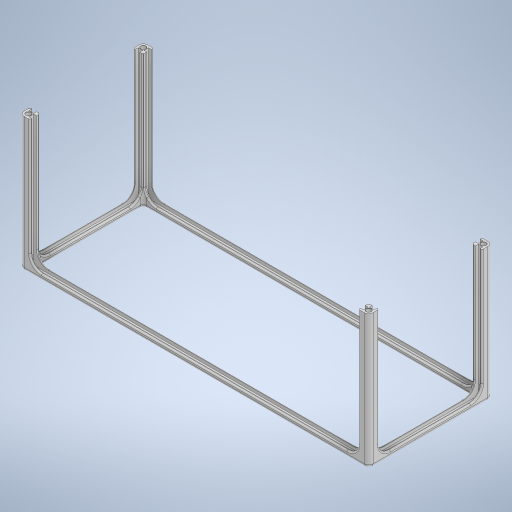
# Autodesk Inventor part: ChamberFrameBottom
Saved by Autodesk Inventor 2023 (Build 270158000, 158)
## iProperties
Created: 2025-11-21
Part Number: ChamberFrameBottom
Material: Generic
Document SubType Name: Modeling
Designer: DanAr
Density: 1 g/cm^3
Appearance: Default
Author: DanAr
Autodesk Inventor part; units mm, degrees
ref_plane "YZ Plane" through (0, 0, 0) normal (1, 0, 0) x (0, 1, 0)
ref_plane "XZ Plane" through (0, 0, 0) normal (0, 1, 0) x (-1, 0, 0)
ref_plane "XY Plane" through (0, 0, 0) normal (0, 0, 1) x (1, 0, 0)
sketch "Sketch1" plane through (0, 0, 0) normal (0, 1, 0) x (-1, 0, 0)
  line L0 (0, 0) -> (234, 0)
  line L1 (234, 0) -> (234, -79)
  line L2 (234, -79) -> (0, -79)
  line L3 (0, -79) -> (0, 0)
  line L4 (2, -77.5) -> (232, -77.5)
  line L5 (232, -77.5) -> (232, -80.5)
  line L6 (232, -80.5) -> (2, -80.5)
  line L7 (2, -80.5) -> (2, -77.5)
  line L8 (2, -77.5) -> (232, -80.5) construction
  line L9 (232, -77.5) -> (2, -80.5) construction
  line L10 (235.5, -2) -> (232.5, -2)
  line L11 (232.5, -2) -> (232.5, -77)
  line L12 (232.5, -77) -> (235.5, -77)
  line L13 (235.5, -77) -> (235.5, -2)
  line L14 (235.5, -2) -> (232.5, -77) construction
  line L15 (232.5, -2) -> (235.5, -77) construction
  line L16 (1.5, -2) -> (-1.5, -2)
  line L17 (-1.5, -2) -> (-1.5, -77)
  line L18 (-1.5, -77) -> (1.5, -77)
  line L19 (1.5, -77) -> (1.5, -2)
  line L20 (1.5, -2) -> (-1.5, -77) construction
  line L21 (-1.5, -2) -> (1.5, -77) construction
  line L22 (2, 1.5) -> (232, 1.5)
  line L23 (232, 1.5) -> (232, -1.5)
  line L24 (232, -1.5) -> (2, -1.5)
  line L25 (2, -1.5) -> (2, 1.5)
  line L26 (2, 1.5) -> (232, -1.5) construction
  line L27 (232, 1.5) -> (2, -1.5) construction
  line L28 (117, 0) -> (117, -79)
  line L29 (231, -3) -> (3, -3)
  line L30 (3, -3) -> (3, -76)
  line L31 (3, -76) -> (231, -76)
  line L32 (231, -76) -> (231, -3)
  line L33 (231, -3) -> (3, -76) construction
  line L34 (3, -3) -> (231, -76) construction
  line L35 (-3, 3) -> (237, 3)
  line L36 (237, 3) -> (237, -82)
  line L37 (237, -82) -> (-3, -82)
  line L38 (-3, -82) -> (-3, 3)
  line L39 (-3, 3) -> (237, -82) construction
  line L40 (237, 3) -> (-3, -82) construction
  point P0 (234, -39.5)
  point P1 (0, -39.5)
  point P2 (117, -39.5)
  dimension "d0" = 79
  dimension "d1" = 234
  dimension "d2" = 230
  dimension "d3" = 3
  dimension "d4" = 75
  dimension "d5" = 3
  dimension "d6" = 75
  dimension "d7" = 3
  dimension "d8" = 230
  dimension "d9" = 3
  dimension "d10" = 73
  dimension "d11" = 228
  dimension "d12" = 240
  dimension "d13" = 85
  constraints: 82 end point, 17 midpoint, 14 parallel, 8 perpendicular, 7 horizontal
  measures "d0" distance of L0.end L1.end
  measures "d1" distance of L1.end L2.end
  measures "d2" distance of L5.end L6.end
  measures "d3" distance of L4.end L5.end
  measures "d4" distance of L12.end L10.start
  measures "d5" distance of L11.end L12.end
  measures "d6" distance of L18.end L16.start
  measures "d7" distance of L17.end L18.end
  measures "d8" horizontal distance of L22.end L24.end
  measures "d9" distance of L22.end L23.end
  measures "d10" distance of L29.end L30.end
  measures "d11" distance of L30.end L31.end
  measures "d12" distance of L36.end L37.end
  measures "d13" distance of L37.end L35.start
extrude "Extrusion1" add sketch "Sketch1" along normal blind 4 contours L0 L25 L24 L28 L29 L30 L31 L4 L7 L2 L3 L18 L19 L16 | L0 L1 L10 L11 L12 L2 L5 L4 L28 L31 L32 L29 L24 L23 | L35 L36 L37 L38
sketch "Sketch2" plane through (0, 0, 0) normal (0, -1, 0) x (1, 0, 0)
  line L0 (3, 3) -> (3, -82) projected
  line L1 (3, -82) -> (-237, -82) projected
  line L2 (3, 3) -> (-237, 3)
  line L3 (-237, 3) -> (-237, -82)
  line L4 (-237, -82) -> (3, -82)
  line L5 (3, -82) -> (3, 3)
  line L6 (-3, -76) -> (-3, -3) projected
  line L7 (-231, -3) -> (-231, -76) projected
  line L8 (-3, -3) -> (-231, -3)
  line L9 (-231, -3) -> (-231, -76)
  line L10 (-231, -76) -> (-3, -76)
  line L11 (-3, -76) -> (-3, -3)
  point P0 (0, 0)
  point P1 (-231, -3)
  point P2 (-3, -76)
  constraints: 16 end point, 4 parallel, 2 horizontal, 2 perpendicular
extrude "Extrusion2" add sketch "Sketch2" against normal blind 2
sketch "Sketch3" plane through (0, 4, 0) normal (0, 1, 0) x (1, 0, 0)
  line L0 (-1.5, 2) -> (-1.5, 77) projected
  line L1 (1.5, 77) -> (1.5, 2) projected
  line L2 (-1.5, 2) -> (1.5, 2)
  line L3 (1.5, 2) -> (1.5, 4)
  line L4 (1.5, 4) -> (-1.5, 4)
  line L5 (-1.5, 4) -> (-1.5, 2)
  line L6 (-232, 1.5) -> (-2, 1.5) projected
  line L7 (-2, -1.5) -> (-232, -1.5) projected
  line L8 (-2, 1.5) -> (-4, 1.5)
  line L9 (-4, 1.5) -> (-4, -1.5)
  line L10 (-4, -1.5) -> (-2, -1.5)
  line L11 (-2, -1.5) -> (-2, 1.5)
  line L12 (-3, 76) -> (-3, 3) projected
  line L13 (-4, 1.5) -> (-3, 1.5)
  line L14 (-3, 3) -> (-4, 3)
  line L15 (-4, 3) -> (-4, 1.5)
  line L16 (-3, 3) -> (-231, 3) projected
  line L17 (-1.5, 3) -> (-1.5, 4)
  line L18 (-1.5, 4) -> (-3, 4)
  line L19 (-3, 4) -> (-3, 3)
  line L20 (-237, -3) -> (3, -3) projected
  line L21 (3, -1.5) -> (3, -3)
  line L22 (3, -3) -> (-4, -3)
  line L23 (-4, -3) -> (-4, -1.5)
  line L24 (1.5, 4) -> (3, 4)
  line L25 (3, 4) -> (3, -1.5)
  line L26 (-1.5, 77) -> (1.5, 77) projected
  line L27 (-1.5, 77) -> (1.5, 77)
  line L28 (1.5, 77) -> (1.5, 75)
  line L29 (1.5, 75) -> (-1.5, 75)
  line L30 (-1.5, 75) -> (-1.5, 77)
  line L31 (-2, 77.5) -> (-232, 77.5) projected
  line L32 (-232, 80.5) -> (-2, 80.5) projected
  line L33 (-2, 77.5) -> (-4, 77.5)
  line L34 (-4, 77.5) -> (-4, 80.5)
  line L35 (-4, 80.5) -> (-2, 80.5)
  line L36 (-2, 80.5) -> (-2, 77.5)
  line L37 (-231, 76) -> (-3, 76) projected
  line L38 (-4, 77.5) -> (-3, 77.5)
  line L39 (-3, 76) -> (-4, 76)
  line L40 (-4, 76) -> (-4, 77.5)
  line L41 (-1.5, 75) -> (-3, 75)
  line L42 (-3, 75) -> (-3, 76)
  line L43 (-1.5, 76) -> (-1.5, 75)
  line L44 (3, 82) -> (-237, 82) projected
  line L45 (1.5, 75) -> (3, 75)
  line L46 (3, 75) -> (3, 82)
  line L47 (3, 82) -> (1.5, 82)
  line L48 (1.5, 82) -> (-4, 82)
  line L49 (-4, 82) -> (-4, 80.5)
  line L50 (-232, 77.5) -> (-230, 77.5)
  line L51 (-230, 77.5) -> (-230, 80.5)
  line L52 (-230, 80.5) -> (-232, 80.5)
  line L53 (-232, 80.5) -> (-232, 77.5)
  line L54 (-235.5, 2) -> (-235.5, 77) projected
  line L55 (-232.5, 77) -> (-232.5, 2) projected
  line L56 (-235.5, 77) -> (-232.5, 77)
  line L57 (-232.5, 77) -> (-232.5, 75)
  line L58 (-232.5, 75) -> (-235.5, 75)
  line L59 (-235.5, 75) -> (-235.5, 77)
  line L60 (-232.5, 75) -> (-231, 75)
  line L61 (-231, 75) -> (-231, 76)
  line L62 (-232.5, 39) -> (-232.5, 75)
  line L63 (-230, 77.5) -> (-231, 77.5)
  line L64 (-231, 76) -> (-230, 76)
  line L65 (-230, 76) -> (-230, 77.5)
  line L66 (-237, 82) -> (-237, -3) projected
  line L67 (-237, 80.5) -> (-237, 82)
  line L68 (-237, 82) -> (-230, 82)
  line L69 (-230, 82) -> (-230, 80.5)
  line L70 (-235.5, 75) -> (-237, 75)
  line L71 (-237, 75) -> (-237, 80.5)
  line L72 (-232.5, 2) -> (-235.5, 2) projected
  line L73 (-232.5, 2) -> (-235.5, 2)
  line L74 (-235.5, 2) -> (-235.5, 4)
  line L75 (-235.5, 4) -> (-232.5, 4)
  line L76 (-232.5, 4) -> (-232.5, 2)
  line L77 (-232, -1.5) -> (-232, 1.5) projected
  line L78 (-232, 1.5) -> (-230, 1.5)
  line L79 (-230, 1.5) -> (-230, -1.5)
  line L80 (-230, -1.5) -> (-232, -1.5)
  line L81 (-232, -1.5) -> (-232, 1.5)
  line L82 (-232.5, 4) -> (-231, 4)
  line L83 (-231, 4) -> (-231, 3)
  line L84 (-232.5, 3) -> (-232.5, 4)
  line L85 (-231, 3) -> (-230, 3)
  line L86 (-230, 3) -> (-230, 1.5)
  line L87 (-230, 1.5) -> (-231, 1.5)
  line L88 (-237, -1.5) -> (-237, -3)
  line L89 (-237, -3) -> (-230, -3)
  line L90 (-230, -3) -> (-230, -1.5)
  line L91 (-235.5, 4) -> (-237, 4)
  line L92 (-237, 4) -> (-237, -1.5)
  point P0 (0, 0)
  point P1 (-2, 80.5)
  point P2 (-1.5, 75)
  point P3 (1.5, 2)
  point P4 (-2, -1.5)
  dimension "d18" = 2
  dimension "d19" = 2
  dimension "d20" = 2
  dimension "d21" = 2
  dimension "d22" = 2
  dimension "d23" = 2
  dimension "d24" = 2
  dimension "d25" = 2
  constraints: 152 end point, 28 parallel, 17 horizontal, 14 perpendicular, 8 point on line
  measures "d18" distance between parallel lines of L2 L4
  measures "d19" distance between parallel lines of L11 L9
  measures "d20" distance between parallel lines of L27 L29
  measures "d21" distance between parallel lines of L36 L34
  measures "d22" distance between parallel lines of L53 L51
  measures "d23" distance between parallel lines of L56 L58
  measures "d24" distance between parallel lines of L72 L75
  measures "d25" distance between parallel lines of L77 L79
extrude "Extrusion3" add sketch "Sketch3" along normal blind 178 contours L2 L1 L24 L25 L21 L20 L23 L7 L11 L6 L15 L14 L12 L18 L0 | L41 L12 L37 L40 L31 L36 L32 L49 L44 L46 L45 L1 L26 L0 | L86 L6 L77 L7 L90 L20 L66 L91 L54 L72 L55 L82 L83 L16 | L37 L61 L60 L55 L56 L54 L70 L66 L44 L69 L32 L53 L31 L65
sketch "Sketch4" plane through (0, 182, 0) normal (0, 1, 0) x (1, 0, 0)
  line L0 (-231, 3) -> (-231, 76) projected
  line L1 (-3, 76) -> (-3, 3) projected
  line L2 (-231, 76) -> (-3, 76)
  line L3 (-3, 76) -> (-3, 3)
  line L4 (-3, 3) -> (-231, 3)
  line L5 (-231, 3) -> (-231, 76)
  line L6 (3, -3) -> (3, 82) projected
  line L7 (-237, 82) -> (-237, -3) projected
  line L8 (3, -3) -> (-237, -3)
  line L9 (-237, -3) -> (-237, 82)
  line L10 (-237, 82) -> (3, 82)
  line L11 (3, 82) -> (3, -3)
  line L12 (-231, 76) -> (-3, 76) projected
  line L13 (-117, 76) -> (-117, 3)
  line L14 (-4, 3) -> (-230, 3) projected
  line L15 (-2, 2) -> (-232, 2)
  line L16 (-232, 2) -> (-232, 77)
  line L17 (-232, 77) -> (-2, 77)
  line L18 (-2, 77) -> (-2, 2)
  line L19 (-2, 2) -> (-232, 77) construction
  line L20 (-232, 2) -> (-2, 77) construction
  point P0 (0, 0)
  point P1 (-117, 39.5)
  point P2 (-231, 3)
  point P3 (-3, 76)
  dimension "d28" = 75
  dimension "d29" = 230
  constraints: 30 end point, 6 parallel, 5 midpoint, 3 horizontal, 3 perpendicular
  measures "d28" distance of L15.end L16.end
  measures "d29" distance of L16.end L17.end
extrude "Extrusion4" add sketch "Sketch4" along normal blind 0.5 contours L15 L16 L17 L18
sketch "Sketch5" plane through (0, 182, 0) normal (0, 1, 0) x (1, 0, 0)
  line L0 (-1.5, 2) -> (-1.5, 4) projected
  line L1 (-1.5, 77) -> (1.5, 77) projected
  line L2 (-1.5, 2) -> (1.5, 2)
  line L3 (1.5, 2) -> (1.5, 77)
  line L4 (1.5, 77) -> (-1.5, 77)
  line L5 (-1.5, 77) -> (-1.5, 2)
  line L6 (-2, 77.5) -> (-232, 77.5) projected
  line L7 (-232, 80.5) -> (-230, 80.5) projected
  line L8 (-2, 77.5) -> (-232, 77.5)
  line L9 (-232, 77.5) -> (-232, 80.5)
  line L10 (-232, 80.5) -> (-2, 80.5)
  line L11 (-2, 80.5) -> (-2, 77.5)
  line L12 (-235.5, 75) -> (-235.5, 77) projected
  line L13 (-232.5, 2) -> (-235.5, 2) projected
  line L14 (-235.5, 77) -> (-232.5, 77)
  line L15 (-232.5, 77) -> (-232.5, 2)
  line L16 (-232.5, 2) -> (-235.5, 2)
  line L17 (-235.5, 2) -> (-235.5, 77)
  line L18 (-232, 1.5) -> (-230, 1.5) projected
  line L19 (-2, 1.5) -> (-2, -1.5) projected
  line L20 (-232, 1.5) -> (-2, 1.5)
  line L21 (-2, 1.5) -> (-2, -1.5)
  line L22 (-2, -1.5) -> (-232, -1.5)
  line L23 (-232, -1.5) -> (-232, 1.5)
  line L24 (-237, -3) -> (3, -3) projected
  line L25 (-230, 82) -> (-237, 82) projected
  line L26 (3, -3) -> (-237, -3)
  line L27 (-237, -3) -> (-237, 82)
  line L28 (-237, 82) -> (3, 82)
  line L29 (3, 82) -> (3, -3)
  line L30 (-2, 77) -> (-232, 77) projected
  line L31 (-2, 2) -> (-2, 77) projected
  line L32 (-232, 77) -> (-2, 77)
  line L33 (-2, 77) -> (-2, 2)
  line L34 (-2, 2) -> (-232, 2)
  line L35 (-232, 2) -> (-232, 77)
  point P0 (0, 0)
  point P1 (-2, 1.5)
  constraints: 48 end point, 12 parallel, 6 horizontal, 6 perpendicular
extrude "Extrusion5" add sketch "Sketch5" along normal blind 2
sketch "Sketch6" plane through (0, 184, 0) normal (0, 1, 0) x (1, 0, 0)
  line L0 (-237, -3) -> (3, -3) projected
  line L1 (-232, 2) -> (-2, 2) projected
  line L2 (3, -3) -> (-2, -3)
  line L3 (-2, -3) -> (-2, 2)
  line L4 (-2, 2) -> (3, 2)
  line L5 (3, 2) -> (3, -3)
  circle A0 centre (0, 0) radius 1.45
  circle A1 centre (0, 79) radius 1.45
  line L6 (-232.5, 2) -> (-235.5, 2) projected
  line L7 (-234, 2) -> (-234, 0)
  line L8 (-234, 0) -> (-234, 79)
  circle A2 centre (-234, 79) radius 1.45
  circle A3 centre (-234, 0) radius 1.45
  line L9 (-237, 82) -> (-237, -3) projected
  line L10 (-234, 0) -> (-237, 0)
  line L11 (-237, 0) -> (-237, -3)
  line L12 (-237, -3) -> (-234, -3)
  line L13 (-234, -3) -> (-234, 0)
  line L14 (0, 79) -> (0, 0)
  dimension "d34" = 2.9
  dimension "d57" = 3
  dimension "d58" = 79
  dimension "d59" = 3
  dimension "d60" = 79
  constraints: 22 end point, 4 centre point, 4 parallel, 3 coincident, 2 horizontal, 2 perpendicular, 2 vertical, 1 midpoint, 1 point on line
  measures "d34" diameter of A0
  measures "d57" distance of L10.end L0.start
  measures "d58" distance of L7.end L8.end
  measures "d59" distance from line of L0 point (0, 0)
  measures "d60" distance of L14.start L14.end
extrude "Extrusion6" cut sketch "Sketch6" against normal blind 20 contours L13 L7 A3 | A3 L10 L13 | A3 L7 L10 | A0 | A1 | A2
fillet "Fillet1" radius 3 4 edges at (-237, 92, 3) (-237, 92, -82) (3, 92, 3) (3, 92, -82)
chamfer "Chamfer1" distance 0.2 angle 45 4 edges at (-235.45, 184, -79) (-235.45, 184, 0) (-1.45, 184, -79) (-1.45, 184, 0)
sketch "Sketch9" plane through (0, 182, 0) normal (0, -1, 0) x (1, 0, 0)
  line L0 (-230, 3) -> (-4, 3) projected
  line L1 (-4, 1.5) -> (-230, 1.5) projected
  line L2 (-230, 3) -> (-4, 3)
  line L3 (-4, 3) -> (-4, 1.5)
  line L4 (-4, 1.5) -> (-230, 1.5)
  line L5 (-230, 1.5) -> (-230, 3)
  line L6 (-4, -1.5) -> (-4, -3) projected
  line L7 (-230, -1.5) -> (-230, -3) projected
  line L8 (-4, -1.5) -> (-230, -1.5)
  line L9 (-230, -1.5) -> (-230, -3)
  line L10 (-230, -3) -> (-4, -3)
  line L11 (-4, -3) -> (-4, -1.5)
  line L12 (-232.5, -4) -> (-231, -4) projected
  line L13 (-231, -75) -> (-232.5, -75) projected
  line L14 (-232.5, -4) -> (-231, -4)
  line L15 (-231, -4) -> (-231, -75)
  line L16 (-231, -75) -> (-232.5, -75)
  line L17 (-232.5, -75) -> (-232.5, -4)
  line L18 (-235.5, -75) -> (-237, -75) projected
  line L19 (-237, -4) -> (-235.5, -4) projected
  line L20 (-235.5, -75) -> (-237, -75)
  line L21 (-237, -75) -> (-237, -4)
  line L22 (-237, -4) -> (-235.5, -4)
  line L23 (-235.5, -4) -> (-235.5, -75)
  line L24 (-230, -77.5) -> (-230, -76) projected
  line L25 (-4, -76) -> (-4, -77.5) projected
  line L26 (-230, -76) -> (-4, -76)
  line L27 (-4, -76) -> (-4, -77.5)
  line L28 (-4, -77.5) -> (-230, -77.5)
  line L29 (-230, -77.5) -> (-230, -76)
  line L30 (-4, -80.5) -> (-4, -82) projected
  line L31 (-230, -82) -> (-230, -80.5) projected
  line L32 (-4, -80.5) -> (-230, -80.5)
  line L33 (-230, -80.5) -> (-230, -82)
  line L34 (-230, -82) -> (-4, -82)
  line L35 (-4, -82) -> (-4, -80.5)
  line L36 (-1.5, -75) -> (-3, -75) projected
  line L37 (-3, -4) -> (-1.5, -4) projected
  line L38 (-3, -75) -> (-1.5, -75)
  line L39 (-1.5, -75) -> (-1.5, -4)
  line L40 (-1.5, -4) -> (-3, -4)
  line L41 (-3, -4) -> (-3, -75)
  line L42 (3, -4) -> (1.5, -4) projected
  line L43 (1.5, -75) -> (3, -75) projected
  line L44 (1.5, -4) -> (3, -4)
  line L45 (3, -4) -> (3, -75)
  line L46 (3, -75) -> (1.5, -75)
  line L47 (1.5, -75) -> (1.5, -4)
  point P0 (0, 0)
  point P1 (-1.5, -75)
  point P2 (-4, -82)
  point P3 (-4, -76)
  point P4 (-4, 3)
  constraints: 64 end point, 16 parallel, 8 horizontal, 8 perpendicular
extrude "Extrusion7" add sketch "Sketch9" along normal blind 2
fillet "Fillet9" radius 2 4 edges at (-3, 91.25, -3) (-3, 91.25, -76) (-231, 91.25, -3) (-231, 91.25, -76)
fillet "Fillet10" radius 3 4 edges at (-232, 183.25, -77) (-232, 183.25, -2) (-2, 183.25, -77) (-2, 183.25, -2)
fillet "Fillet11" radius 8 16 edges at (-4, 4, -76.616) (-4, 4, -81.25) (2.25, 4, -4) (-2.384, 4, -4) (-4, 4, -2.384) (-4, 4, 2.25) (-2.384, 4, -75) (2.25, 4, -75) (-230, 4, -81.25) (-230, 4, -76.616) (-231.616, 4, -75) (-236.25, 4, -75) (-231.616, 4, -4) (-236.25, 4, -4) (-230, 4, -2.384) (-230, 4, 2.25)
fillet "Fillet12" radius 2 16 edges at (2.25, 180, -75) (-2.384, 180, -75) (2.25, 180, -4) (-2.384, 180, -4) (-4, 180, 2.25) (-4, 180, -2.384) (-231.616, 180, -4) (-236.25, 180, -4) (-230, 180, 2.25) (-230, 180, -2.384) (-236.25, 180, -75) (-231.616, 180, -75) (-230, 180, -76.616) (-230, 180, -81.25) (-4, 180, -76.616) (-4, 180, -81.25)
fillet "Fillet13" radius 3 8 edges at (-234, 2, -77) (-232, 2, -79) (-234, 2, -2) (-232, 2, 0) (0, 2, -77) (-2, 2, -79) (0, 2, -2) (-2, 2, 0)
fillet "Fillet14" radius 2 16 edges at (-117, 0, 3) (2.1213, 0, 2.1213) (3, 0, -39.5) (2.1213, 0, -81.1213) (-117, 0, -82) (-236.1213, 0, -81.1213) (-237, 0, -39.5) (-236.1213, 0, 2.1213) (-3.5858, 0, -3.5858) (-117, 0, -3) (-230.4142, 0, -3.5858) (-231, 0, -39.5) (-230.4142, 0, -75.4142) (-117, 0, -76) (-3.5858, 0, -75.4142) (-3, 0, -39.5)
fillet "Fillet15" radius 1 80 edges at (-230.8535, 10.0213, -74.7514) (-231, 5.1086, -71.063) (-231, 4, -39.5) (-231, 5.1086, -7.937) (-230.8536, 10.0204, -4.2488) (-230.7321, 95, -4) (-230.8537, 178.9669, -4.2493) (-231, 179.9319, -5.4824) (-231, 180, -39.5) (-231, 179.9319, -73.5176) (-230.8537, 178.9669, -74.7507) (-230.7321, 95, -75) (-226.063, 5.1086, -76) (-117, 4, -76) (-7.937, 5.1086, -76) (-4.2486, 10.0213, -75.8535) (-4, 95, -75.7321) (-4.2493, 178.9669, -75.8537) (-5.4824, 179.9319, -76) (-117, 180, -76) (-228.5176, 179.9319, -76) (-229.7507, 178.9669, -75.8538) (-230, 95, -75.7321) (-229.7512, 10.0204, -75.8536) (-237, 4, -39.5) (-237, 6.3431, -6.3431) (-237, 95, -4) (-237, 179.4142, -4.5858) (-237, 180, -39.5) (-237, 179.4142, -74.4142) (-237, 95, -75) (-237, 6.3431, -72.6569) (-230, 95, -82) (-229.4142, 179.4142, -82) (-117, 180, -82) (-4.5858, 179.4142, -82) (-4, 95, -82) (-6.3431, 6.3431, -82) (-117, 4, -82) (-227.6569, 6.3431, -82) (-226.063, 5.1086, -3) (-229.7514, 10.0213, -3.1465) (-230, 95, -3.2679) (-229.7507, 178.9669, -3.1463) (-228.5176, 179.9319, -3) (-117, 180, -3) (-5.4824, 179.9319, -3) (-4.2493, 178.9669, -3.1463) (-4, 95, -3.2679) (-4.2486, 10.0213, -3.1465) (-7.937, 5.1086, -3) (-117, 4, -3) (-6.3431, 6.3431, 3) (-4, 95, 3) (-4.5858, 179.4142, 3) (-117, 180, 3) (-229.4142, 179.4142, 3) (-230, 95, 3) (-227.6569, 6.3431, 3) (-117, 4, 3) (-3, 5.1086, -7.937) (-3.1464, 10.0204, -4.2488) (-3.2679, 95, -4) (-3.1463, 178.9669, -4.2493) (-3, 179.9319, -5.4824) (-3, 180, -39.5) (-3, 179.9319, -73.5176) (-3.1462, 178.9669, -74.7507) (-3.2679, 95, -75) (-3.1464, 10.0204, -74.7512) (-3, 5.1086, -71.063) (-3, 4, -39.5) (3, 6.3431, -72.6569) (3, 95, -75) (3, 179.4142, -74.4142) (3, 180, -39.5) (3, 179.4142, -4.5858) (3, 95, -4) (3, 6.3431, -6.3431) (3, 4, -39.5)
sketch "Sketch10" plane through (0, 184, 0) normal (0, 1, 0) x (1, 0, 0)
  line L0 (-12, -1.5) -> (-222, -1.5) projected
  line L1 (-117, -1.5) -> (-117, 1.5)
  line L2 (-222, 1.5) -> (-12, 1.5) projected
  line L3 (-232, -1.6) -> (-2, -1.6)
  line L4 (-2, -1.6) -> (-2, 1.6)
  line L5 (-2, 1.6) -> (-232, 1.6)
  line L6 (-232, 1.6) -> (-232, -1.6)
  line L7 (-232, -1.6) -> (-2, 1.6) construction
  line L8 (-2, -1.6) -> (-232, 1.6) construction
  line L9 (-235.5, 5) -> (-235.5, 74) projected
  line L10 (-235.5, 39.5) -> (-232.5, 39.5)
  line L11 (-232.5, 74) -> (-232.5, 5) projected
  line L12 (-235.6, 77) -> (-232.4, 77)
  line L13 (-232.4, 77) -> (-232.4, 2)
  line L14 (-232.4, 2) -> (-235.6, 2)
  line L15 (-235.6, 2) -> (-235.6, 77)
  line L16 (-235.6, 77) -> (-232.4, 2) construction
  line L17 (-232.4, 77) -> (-235.6, 2) construction
  line L18 (-117, 1.5) -> (-117, 78)
  line L19 (-229, 78) -> (-5, 78) projected
  line L20 (-117, 78) -> (-117, 80.5)
  line L21 (-222, 80.5) -> (-12, 80.5) projected
  line L22 (-228, 77.5) -> (-6, 77.5) projected
  line L23 (-117, 77.5) -> (-117, 80.5)
  line L24 (-232, 77.4) -> (-2, 77.4)
  line L25 (-2, 77.4) -> (-2, 80.6)
  line L26 (-2, 80.6) -> (-232, 80.6)
  line L27 (-232, 80.6) -> (-232, 77.4)
  line L28 (-232, 77.4) -> (-2, 80.6) construction
  line L29 (-2, 77.4) -> (-232, 80.6) construction
  line L30 (-1.5, 5) -> (-1.5, 74) projected
  line L31 (-1.5, 39.5) -> (1.5, 39.5)
  line L32 (1.5, 67) -> (1.5, 12) projected
  line L33 (1.6, 2) -> (-1.6, 2)
  line L34 (-1.6, 2) -> (-1.6, 77)
  line L35 (-1.6, 77) -> (1.6, 77)
  line L36 (1.6, 77) -> (1.6, 2)
  line L37 (1.6, 2) -> (-1.6, 77) construction
  line L38 (-1.6, 2) -> (1.6, 77) construction
  point P0 (0, 0)
  point P1 (-117, 0)
  point P2 (-234, 39.5)
  point P3 (-117, 79)
  point P4 (0, 39.5)
  dimension "d61" = 3.2
  dimension "d62" = 3.2
  dimension "d63" = 3.2
  dimension "d64" = 3.2
  constraints: 60 end point, 21 midpoint, 8 parallel, 5 perpendicular, 4 horizontal
  measures "d61" distance of L3.end L4.end
  measures "d62" distance of L13.end L14.end
  measures "d63" distance of L24.end L25.end
  measures "d64" distance of L34.end L35.end
extrude "Extrusion8" cut sketch "Sketch10" against normal up to surface (182 mm away)
fillet "Fillet16" radius 3 8 edges at (0, 2, -77) (-2, 2, -79) (0, 2, -2) (-2, 2, 0) (-232, 2, 0) (-234, 2, -2) (-234, 2, -77) (-232, 2, -79)
sketch "Sketch14" plane through (3, 184, 0) normal (1, 0, 0) x (0, 0, -1)
  line L0 (-3, -182) -> (-3, 0) projected
  line L1 (82, 0) -> (82, -182) projected
  line L2 (-3, 0) -> (82, 0)
  line L3 (82, 0) -> (82, -91)
  line L4 (82, -91) -> (-3, -91)
  line L5 (-3, -91) -> (-3, 0)
  line L6 (39.5, -91) -> (94.1389, -91)
  line L7 (94.1389, -91) -> (94.1389, -195.5904)
  line L8 (94.1389, -195.5904) -> (39.5, -195.5904)
  line L9 (39.5, -195.5904) -> (39.5, -91)
  point P0 (0, -184)
  point P1 (-3, -91)
  constraints: 16 end point, 4 parallel, 2 horizontal, 2 midpoint, 2 perpendicular
extrude "Extrusion9" cut sketch "Sketch14" against normal blind 244
sketch "Sketch15" plane through (-234, 2, 3) normal (0, 0, 1) x (1, 0, 0)
  line L0 (-3, 10) -> (-3, 91) projected
  line L1 (0, -2) -> (234, -2) projected
  line L2 (-3, 91) -> (117, 91)
  line L3 (117, 91) -> (117, -2)
  line L4 (117, -2) -> (-3, -2)
  line L5 (-3, -2) -> (-3, 91)
  line L6 (117, 91) -> (237, 91)
  line L7 (237, 91) -> (237, -2)
  line L8 (237, -2) -> (117, -2)
  line L9 (117, -2) -> (117, 91)
  constraints: 16 end point, 4 parallel, 2 horizontal, 2 perpendicular, 1 midpoint, 1 point on line
extrude "Extrusion10" cut sketch "Sketch15" against normal blind 244 contours L0 L2 L3 L1 L4 L5
sketch "Sketch23" plane through (3, 93, 0) normal (0, 1, 0) x (1, 0, 0)
  circle A0 centre (-3, 0) radius 1.6
  dimension "d101" = 3.2
  constraints: 1 centre point, 1 coincident
  measures "d101" diameter of A0
extrude "Extrusion17" cut sketch "Sketch23" against normal blind 13
fillet "Fillet22" radius 0.2 1 edges at (-1.6, 93, 0)
fillet "Fillet23" radius 1 1 edges at (-1.6, 80, 0)
sketch "Sketch25" plane through (3, 2, 0) normal (1, 0, 0) x (0, 0, -1)
  line L0 (-3, 10) -> (-3, 91) projected
  line L1 (4, 91) -> (4, 10) projected
  line L2 (-3, 91) -> (4, 91)
  line L3 (4, 91) -> (4, 90)
  line L4 (4, 90) -> (-3, 90)
  line L5 (-3, 90) -> (-3, 91)
  point P0 (0, -2)
  dimension "d107" = 1
  constraints: 8 end point, 2 parallel, 1 horizontal, 1 perpendicular, 1 point on line
  measures "d107" distance between parallel lines of L2 L4
extrude "Extrusion18" cut sketch "Sketch25" against normal blind 13
fillet "Fillet25" radius 0.2 1 edges at (-1.6, 92, 0)
mirror "Mirror1" about plane through (-117, 93, 3) normal (-1, 0, 0)
mirror "Mirror2" about plane through (3, -11.5904, -39.5) normal (0, 0, -1)
body "Solid1"
